Autodesk Fusion 360 part; units mm, degrees
(part 2 of 4)
sketch "Sketch1 (2)" plane through (0, -3.5, 0) normal (0, -1, 0) x (1, 0, 0) in component "Bay Cover"
  line L0 (0, -59.2) -> (2.1078, -61.3078)
  line L1 (2.1078, -61.3078) -> (5.9078, -61.3078)
  line L2 (5.9078, -61.3078) -> (9.8, -65.2)
  line L3 (9.8, -65.2) -> (18.2, -65.2)
  line L4 (18.2, -65.2) -> (23.2, -60.2)
  line L5 (23.2, -60.2) -> (87.3, -60.2)
  line L6 (87.3, -60.2) -> (92.3, -65.2)
  line L7 (92.3, -65.2) -> (100.7, -65.2)
  line L8 (100.7, -65.2) -> (108.2, -57.7)
  line L9 (108.2, -57.7) -> (108.2, 57.7)
  line L10 (108.2, 57.7) -> (100.7, 65.2)
  line L11 (100.7, 65.2) -> (92.3, 65.2)
  line L12 (92.3, 65.2) -> (87.3, 60.2)
  line L13 (87.3, 60.2) -> (23.2, 60.2)
  line L14 (23.2, 60.2) -> (18.2, 65.2)
  line L15 (18.2, 65.2) -> (9.8, 65.2)
  line L16 (9.8, 65.2) -> (5.9078, 61.3078)
  line L17 (5.9078, 61.3078) -> (2.1078, 61.3078)
  line L18 (2.1078, 61.3078) -> (0, 59.2)
  line L19 (0, 59.2) -> (0, 55.2)
  line L20 (0, 55.2) -> (4.8, 55.2)
  line L21 (4.8, 55.2) -> (4.8, 57.3078)
  line L22 (4.8, 57.3078) -> (9.5424, 55.2)
  line L23 (9.5424, 55.2) -> (100.0828, 55.2)
  line L24 (100.0828, 55.2) -> (103.2, 52.0828)
  line L25 (103.2, 52.0828) -> (103.2, -52.0828)
  line L26 (103.2, -52.0828) -> (100.0828, -55.2)
  line L27 (100.0828, -55.2) -> (9.5424, -55.2)
  line L28 (9.5424, -55.2) -> (4.8, -57.3078)
  line L29 (4.8, -57.3078) -> (4.8, -55.2)
  line L30 (4.8, -55.2) -> (0, -55.2)
  line L31 (0, -55.2) -> (0, -59.2)
  circle A0 centre (14, -60.2) radius 2.25
  circle A1 centre (96.5, -60.2) radius 2.25
  circle A2 centre (14, 60.2) radius 2.25
  circle A3 centre (96.5, 60.2) radius 2.25
  line L32 (4.8, 55.2) -> (0, 55.2)
  line L33 (0, 55.2) -> (0, 52)
  line L34 (0, 52) -> (100, 52)
  line L35 (100, 52) -> (100, -52)
  line L36 (100, -52) -> (0, -52)
  line L37 (0, -52) -> (0, -55.2)
  line L38 (0, -55.2) -> (4.8, -55.2)
  line L39 (4.8, -55.2) -> (4.8, -57.3078)
  line L40 (4.8, -57.3078) -> (9.5424, -55.2)
  line L41 (9.5424, -55.2) -> (100.0828, -55.2)
  line L42 (100.0828, -55.2) -> (103.2, -52.0828)
  line L43 (103.2, -52.0828) -> (103.2, 52.0828)
  line L44 (103.2, 52.0828) -> (100.0828, 55.2)
  line L45 (100.0828, 55.2) -> (9.5424, 55.2)
  line L46 (9.5424, 55.2) -> (4.8, 57.3078)
  line L47 (4.8, 57.3078) -> (4.8, 55.2)
extrude "Extrude1''''" add sketch "Sketch1 (2)" along normal blind 2 separate body makes body 5 in component "Bay Cover"
sketch "Sketch1 (3)" plane through (0, -5.5, 0) normal (0, -1, 0) x (1, 0, 0) in component "Spacer 40 mm"
  circle A0 centre (96.5, -60.2) radius 2.25
  circle A1 centre (14, -60.2) radius 2.25
  circle A2 centre (96.5, 60.2) radius 2.25
  circle A3 centre (14, 60.2) radius 2.25
  line L0 (0, -52) -> (0, -59.2)
  line L1 (0, -59.2) -> (2.1078, -61.3078)
  line L2 (2.1078, -61.3078) -> (5.9078, -61.3078)
  line L3 (5.9078, -61.3078) -> (9.8, -65.2)
  line L4 (9.8, -65.2) -> (18.2, -65.2)
  line L5 (18.2, -65.2) -> (23.2, -60.2)
  line L6 (23.2, -60.2) -> (87.3, -60.2)
  line L7 (87.3, -60.2) -> (92.3, -65.2)
  line L8 (92.3, -65.2) -> (100.7, -65.2)
  line L9 (100.7, -65.2) -> (108.2, -57.7)
  line L10 (108.2, -57.7) -> (108.2, 57.7)
  line L11 (108.2, 57.7) -> (100.7, 65.2)
  line L12 (100.7, 65.2) -> (92.3, 65.2)
  line L13 (92.3, 65.2) -> (87.3, 60.2)
  line L14 (87.3, 60.2) -> (23.2, 60.2)
  line L15 (23.2, 60.2) -> (18.2, 65.2)
  line L16 (18.2, 65.2) -> (9.8, 65.2)
  line L17 (9.8, 65.2) -> (5.9078, 61.3078)
  line L18 (5.9078, 61.3078) -> (2.1078, 61.3078)
  line L19 (2.1078, 61.3078) -> (0, 59.2)
  line L20 (0, 59.2) -> (0, 52)
  line L21 (0, 52) -> (100, 52)
  line L22 (100, 52) -> (100, -52)
  line L23 (100, -52) -> (0, -52)
  circle A4 centre (14, 60.2) radius 2.25
  circle A5 centre (14, 60.2) radius 4.25
  dimension "d114" = 8.5
  constraint concentric A3 A4
  constraint concentric A4 A5
  measures "d114" diameter of A5
extrude "Extrude1'''''" add sketch "Sketch1 (3)" along normal blind 40 separate body contours A5 makes body 6 in component "Spacer 40 mm"
sketch "Sketch2" plane through (0, -5.5, 0) normal (0, -1, 0) x (1, 0, 0) in component "Spacer 40 mm"
  circle A0 centre (96.5, -60.2) radius 2.25
  circle A1 centre (14, -60.2) radius 2.25
  circle A2 centre (96.5, 60.2) radius 2.25
  circle A3 centre (14, 60.2) radius 2.25
  line L0 (0, -52) -> (0, -59.2)
  line L1 (0, -59.2) -> (2.1078, -61.3078)
  line L2 (2.1078, -61.3078) -> (5.9078, -61.3078)
  line L3 (5.9078, -61.3078) -> (9.8, -65.2)
  line L4 (9.8, -65.2) -> (18.2, -65.2)
  line L5 (18.2, -65.2) -> (23.2, -60.2)
  line L6 (23.2, -60.2) -> (87.3, -60.2)
  line L7 (87.3, -60.2) -> (92.3, -65.2)
  line L8 (92.3, -65.2) -> (100.7, -65.2)
  line L9 (100.7, -65.2) -> (108.2, -57.7)
  line L10 (108.2, -57.7) -> (108.2, 57.7)
  line L11 (108.2, 57.7) -> (100.7, 65.2)
  line L12 (100.7, 65.2) -> (92.3, 65.2)
  line L13 (92.3, 65.2) -> (87.3, 60.2)
  line L14 (87.3, 60.2) -> (23.2, 60.2)
  line L15 (23.2, 60.2) -> (18.2, 65.2)
  line L16 (18.2, 65.2) -> (9.8, 65.2)
  line L17 (9.8, 65.2) -> (5.9078, 61.3078)
  line L18 (5.9078, 61.3078) -> (2.1078, 61.3078)
  line L19 (2.1078, 61.3078) -> (0, 59.2)
  line L20 (0, 59.2) -> (0, 52)
  line L21 (0, 52) -> (100, 52)
  line L22 (100, 52) -> (100, -52)
  line L23 (100, -52) -> (0, -52)
  line L24 (14, 60.2) -> (14, 65.2) construction
  circle A4 centre (14, 60.2) radius 4.25 construction
  line L25 (14, 65.2) -> (14, 64.45) construction
  dimension "d117" = 0.75
  constraint coincident A3.centre L24.start
  constraint midpoint L16 L24.end
  constraint coincident A4 L25.end
  constraint coincident L24 L25.end
  measures "d117" distance of L24.end L25.end
sketch "More Fill Ins" plane through (0, 7, 0) normal (0, 1, 0) x (-1, 0, 0) in component "End Frame A"
  line L0 (-26.9133, 50.2) -> (-55.25, 8.8457)
  line L1 (-55.25, 8.8457) -> (-83.5867, 50.2)
  line L2 (-83.5867, 50.2) -> (-26.9133, 50.2)
  line L3 (-61.3112, 0) -> (-95.709, -50.2)
  line L4 (-95.709, -50.2) -> (-98.2, -50.2)
  line L5 (-98.2, -50.2) -> (-98.2, 50.2)
  line L6 (-98.2, 50.2) -> (-95.709, 50.2)
  line L7 (-95.709, 50.2) -> (-61.3112, 0)
  line L8 (-14.791, -50.2) -> (-49.1888, 0)
  line L9 (-49.1888, 0) -> (-14.791, 50.2)
  line L10 (-14.791, 50.2) -> (-12.3, 50.2)
  line L11 (-12.3, 50.2) -> (-12.3, -50.2)
  line L12 (-12.3, -50.2) -> (-14.791, -50.2)
  line L13 (-26.9133, -50.2) -> (-83.5867, -50.2)
  line L14 (-83.5867, -50.2) -> (-55.25, -8.8457)
  line L15 (-55.25, -8.8457) -> (-26.9133, -50.2)
  circle A0 centre (-14, -60.2) radius 1.5
  circle A1 centre (-14, 60.2) radius 1.5
  circle A2 centre (-96.5, -60.2) radius 1.5
  circle A3 centre (-96.5, 60.2) radius 1.5
  line L16 (-104.0433, 68.7355) -> (-105.0433, 67.7355)
  line L17 (-105.0433, 67.7355) -> (-105.0433, 60.8567)
  line L18 (-105.0433, 60.8567) -> (-108.2, 57.7)
  line L19 (-108.2, 57.7) -> (-108.2, -57.7)
  line L20 (-108.2, -57.7) -> (-100.7, -65.2)
  line L21 (-100.7, -65.2) -> (-92.3, -65.2)
  line L22 (-92.3, -65.2) -> (-87.3, -60.2)
  line L23 (-87.3, -60.2) -> (-23.2, -60.2)
  line L24 (-23.2, -60.2) -> (-18.2, -65.2)
  line L25 (-18.2, -65.2) -> (-9.8, -65.2)
  line L26 (-9.8, -65.2) -> (-2.3, -57.7)
  line L27 (-2.3, -57.7) -> (-2.3, 57.7)
  line L28 (-2.3, 57.7) -> (-5.4567, 60.8567)
  line L29 (-5.4567, 60.8567) -> (-5.4567, 67.7355)
  line L30 (-5.4567, 67.7355) -> (-6.4567, 68.7355)
  line L31 (-6.4567, 68.7355) -> (-8.2145, 68.7355)
  line L32 (-8.2145, 68.7355) -> (-11.75, 65.2)
  line L33 (-11.75, 65.2) -> (-16.25, 65.2)
  line L34 (-16.25, 65.2) -> (-19.7855, 68.7355)
  line L35 (-19.7855, 68.7355) -> (-21.5433, 68.7355)
  line L36 (-21.5433, 68.7355) -> (-22.5433, 67.7355)
  line L37 (-22.5433, 67.7355) -> (-22.5433, 60.8567)
  line L38 (-22.5433, 60.8567) -> (-23.2, 60.2)
  line L39 (-23.2, 60.2) -> (-87.3, 60.2)
  line L40 (-87.3, 60.2) -> (-87.9567, 60.8567)
  line L41 (-87.9567, 60.8567) -> (-87.9567, 67.7355)
  line L42 (-87.9567, 67.7355) -> (-88.9567, 68.7355)
  line L43 (-88.9567, 68.7355) -> (-90.7145, 68.7355)
  line L44 (-90.7145, 68.7355) -> (-94.25, 65.2)
  line L45 (-94.25, 65.2) -> (-98.75, 65.2)
  line L46 (-98.75, 65.2) -> (-102.2855, 68.7355)
  line L47 (-102.2855, 68.7355) -> (-104.0433, 68.7355)
  line L48 (-102.2855, 68.7355) -> (-90.7145, 68.7355)
  line L49 (-19.7855, 68.7355) -> (-8.2145, 68.7355)
  line L50 (-98.2, -45.8964) -> (-92.7601, -45.8964)
  line L51 (-17.7399, -45.8964) -> (-12.3, -45.8964)
  constraint coincident L46.end L47.start
  constraint coincident L43.end L44.start
  constraint coincident L34.end L35.start
  constraint coincident L31.end L32.start
  constraint coincident L5 L50.start
  constraint coincident L3 L50.end
  constraint perpendicular L5 L50
  constraint coincident L8 L51.start
  constraint coincident L11 L51.end
  constraint perpendicular L11 L51
extrude "Extrude8" add sketch "More Fill Ins" against normal blind 3 contours L3 L4 L5 L50 | L8 L11 L12 L51 | L44 L45 L46 L48 | L32 L33 L34 L49 bodies 3 in component "End Frame A"
extrude "Extrude3''" add 1 faces at (14.3152, 9, 61.4563) along direction (0, 1, 0) blind 1 on bodies 4 bodies 4 in component "Standoff for End Frame"
extrude "Extrude9" add 4 faces at (20.0096, -1, 67.1211) (102.5096, -1, 67.1211) (19.9406, -1, -53.3479) (90.5594, -1, -53.3479) along direction (0, -1, 0) blind 9 on bodies 3 bodies 3 in component "End Frame A"
ref_plane "WorkPlane1" through (14, 4, 60.2) normal (1, 0, 0) x (0, 1, 0) in component "End Frame A"
sketch "Sketch8" plane through (14, 4, 60.2) normal (1, 0, 0) x (0, 1, 0) in component "End Frame A"
  line L0 (0, -4.2) -> (0, 0)
  line L1 (0, 0) -> (-14, 0)
  line L2 (-14, 0) -> (-14, -4.2)
  line L3 (-14, 0) -> (0, 0)
  line L4 (0, -117.9) -> (0, -2.5)
  line L5 (0, -2.5) -> (3, -2.5)
  line L6 (3, -2.5) -> (3, -117.9)
  line L7 (3, -117.9) -> (0, -117.9)
  line L8 (0, -124.6) -> (0, -120.4)
  line L9 (0, -120.4) -> (-14, -120.4)
  line L10 (-14, -120.4) -> (-14, -124.6)
  line L11 (-14, -120.4) -> (0, -120.4)
  line L12 (0, -125.4) -> (0, -117.9)
  line L13 (0, -117.9) -> (3, -117.9)
  line L14 (3, -117.9) -> (3, -125.4)
  line L15 (3, -125.4) -> (0, -125.4)
  line L16 (-14, -4.2) -> (0, -9.6008)
  line L17 (-14, -124.6) -> (-11.1871, -125.4)
  line L18 (-11.1871, -125.4) -> (0, -125.4)
  line L19 (-14, -124.6) -> (-14, -123.6)
  line L20 (-14, -123.6) -> (0, -123.6)
  line L21 (0, -125.4) -> (0, -123.6)
  line L22 (-14, -4.2) -> (-14, -3.2)
  line L23 (-14, -3.2) -> (0, -3.2)
  dimension "d124" = 1
  dimension "d125" = 90
  dimension "d126" = 180
  dimension "d127" = 1
  constraint coincident L2.end L16.start
  constraint coincident L4 L16.end
  constraint coincident L10.end L17.start
  constraint coincident L12.start L15.end
  constraint perpendicular L12 L18
  constraint parallel L10 L19
  constraint coincident L12 L20.end
  constraint horizontal L23
  constraint coincident L4 L23.end
  measures "d124" distance of L10.end L19.end
  measures "d125" angle of L19 L20
  measures "d126" angle of L21 L22
  measures "d127" distance of L2.end L22.end
extrude "Extrude10" add sketch "Sketch8" along normal mid plane 2 contours L0 L2 L4 L16 L22 L23 | L8 L10 L12 L17 L18 L19 L20 L21 bodies 3 in component "End Frame A"
ref_plane "WorkPlane2" through (96.5, -10, -60.2) normal (-1, 0, 0) x (0, -1, 0) in component "End Frame A"
sketch "Sketch9" plane through (96.5, -10, -60.2) normal (-1, 0, 0) x (0, 1, 0) in component "End Frame A"
  line L0 (14, -116.3208) -> (0, -116.3208)
  line L1 (0, -116.3208) -> (0, -116.2)
  line L2 (0, -116.2) -> (14, -110.7992)
  line L3 (14, -110.7992) -> (14, -116.3208)
  line L4 (14, 4.0792) -> (0, 4.0792)
  line L5 (0, 4.0792) -> (0, 4.2)
  line L6 (0, 4.2) -> (2.8129, 5)
  line L7 (2.8129, 5) -> (14, 5)
  line L8 (14, 5) -> (14, 4.0792)
  line L9 (14, 5) -> (2.8129, 5)
  line L10 (2.8129, 5) -> (0, 4.2)
  line L11 (0, 4.2) -> (0, 3.2)
  line L12 (0, 3.2) -> (14, 3.2)
  line L13 (14, 3.2) -> (14, 5)
  line L14 (14, -110.7992) -> (0, -116.2)
  line L15 (0, -116.2) -> (0, -117.2)
  line L16 (0, -117.2) -> (14, -117.2)
  line L17 (14, -117.2) -> (14, -110.7992)
  dimension "d130" = 1
  dimension "d131" = 1
  constraint coincident L7.end L8.start
  constraint coincident L6.end L7.start
  constraint coincident L5.end L6.start
  constraint perpendicular L4 L11
  constraint perpendicular L8 L12
  constraint perpendicular L9 L13
  constraint coincident L2.end L3.start
  constraint coincident L1.end L2.start
  constraint perpendicular L0 L15
  constraint perpendicular L3 L16
  constraint perpendicular L16 L17
  measures "d130" distance of L5.end L11.end
  measures "d131" distance of L1.end L15.end
extrude "Extrude11" add sketch "Sketch9" along normal mid plane 2 bodies 3 in component "End Frame A"
sketch "Mounts" plane through (0, -10, 0) normal (0, -1, 0) x (1, 0, 0) in component "End Frame B"
  arc A0 (97.5, 56.1208) -> (100.7, 60.2) centre (96.5, 60.2) ccw
  arc A1 (94.25, 60.2) -> (98.75, 60.2) centre (96.5, 60.2) ccw
  line L0 (88.4567, 68.2355) -> (92.3, 64.3923)
  line L1 (92.3, 64.3923) -> (92.3, 60.2)
  arc A2 (92.3, 60.2) -> (95.5, 56.1208) centre (96.5, 60.2) ccw
  line L2 (95.5, 56.1208) -> (95.5, 56)
  line L3 (95.5, 56) -> (97.5, 56)
  line L4 (97.5, 56) -> (97.5, 56.1208)
  line L5 (91.5, 57.95) -> (87.9645, 54.4145)
  line L6 (87.9645, 52.6567) -> (88.4645, 52.1567)
  line L7 (87.9645, 52.6567) -> (87.9645, 54.4145)
  line L8 (88.4645, 52.1567) -> (92.3077, 56)
  line L9 (91.5, 57.95) -> (96.5, 57.95)
  line L10 (91.5, 62.45) -> (96.5, 62.45)
  line L11 (88.4645, 68.2433) -> (87.9645, 67.7433)
  line L12 (87.9645, 67.7433) -> (87.9645, 65.9855)
  line L13 (87.9645, 65.9855) -> (91.5, 62.45)
  line L14 (92.3077, 64.4) -> (96.5, 64.4)
  line L15 (92.3077, 56) -> (96.5, 56)
  circle A3 centre (96.5, 60.2) radius 2.25
  circle A4 centre (96.5, 60.2) radius 4.2
  line L16 (92.3077, 64.4) -> (88.4567, 68.2355)
  circle A5 centre (14, 60.2) radius 1.5
  circle A6 centre (96.5, -60.2) radius 1.5
  line L17 (9.8077, 64.4) -> (5.9567, 68.2355)
  line L18 (5.9645, 68.2433) -> (5.4645, 67.7433)
  line L19 (5.4645, 67.7433) -> (5.4645, 65.9855)
  line L20 (5.4645, 65.9855) -> (9, 62.45)
  line L21 (9.8077, 64.4) -> (14, 64.4)
  circle A7 centre (14, 60.2) radius 4.2
  line L22 (9, 62.45) -> (14, 62.45)
  circle A8 centre (14, 60.2) radius 2.25
  line L23 (9, 57.95) -> (14, 57.95)
  line L24 (9.8077, 56) -> (14, 56)
  line L25 (5.9645, 52.1567) -> (9.8077, 56)
  line L26 (9, 57.95) -> (5.4645, 54.4145)
  line L27 (5.4645, 52.6567) -> (5.4645, 54.4145)
  line L28 (5.4645, 52.6567) -> (5.9645, 52.1567)
  line L29 (92.3077, -56) -> (88.4567, -52.1645)
  line L30 (88.4645, -52.1567) -> (87.9645, -52.6567)
  line L31 (87.9645, -52.6567) -> (87.9645, -54.4145)
  line L32 (87.9645, -54.4145) -> (91.5, -57.95)
  line L33 (92.3077, -56) -> (96.5, -56)
  circle A9 centre (96.5, -60.2) radius 4.2
  line L34 (91.5, -57.95) -> (96.5, -57.95)
  circle A10 centre (96.5, -60.2) radius 2.25
  line L35 (91.5, -62.45) -> (96.5, -62.45)
  line L36 (92.3077, -64.4) -> (96.5, -64.4)
  line L37 (88.4645, -68.2433) -> (92.3077, -64.4)
  line L38 (91.5, -62.45) -> (87.9645, -65.9855)
  line L39 (87.9645, -67.7433) -> (87.9645, -65.9855)
  line L40 (87.9645, -67.7433) -> (88.4645, -68.2433)
  line L41 (9.8077, -56) -> (5.9567, -52.1645)
  line L42 (5.9645, -52.1567) -> (5.4645, -52.6567)
  line L43 (5.4645, -52.6567) -> (5.4645, -54.4145)
  line L44 (5.4645, -54.4145) -> (9, -57.95)
  line L45 (9.8077, -56) -> (14, -56)
  circle A11 centre (14, -60.2) radius 4.2
  line L46 (9, -57.95) -> (14, -57.95)
  circle A12 centre (14, -60.2) radius 2.25
  line L47 (9, -62.45) -> (14, -62.45)
  line L48 (9.8077, -64.4) -> (14, -64.4)
  line L49 (5.9645, -68.2433) -> (9.8077, -64.4)
  line L50 (9, -62.45) -> (5.4645, -65.9855)
  line L51 (5.4645, -67.7433) -> (5.4645, -65.9855)
  line L52 (5.4645, -67.7433) -> (5.9645, -68.2433)
  dimension "d138" = -82.5
  dimension "d139" = -120.4
  constraint concentric A0 A3
  constraint coincident L1.end A4
  constraint coincident L0.start L16.end
extrude "Extrude1''''''" add sketch "Mounts" against normal blind 17 separate body contours A0 A1 A2 L9 L10 A3 A4 | L0 L1 L10 L14 A4 L16 | A2 L2 L5 L6 L7 L8 L9 L15 A4 | L0 L1 L10 L11 L12 L13 | L17 L18 L19 L20 L21 A7 L22 | A7 L22 A8 L23 | A7 L23 L24 L25 L26 L27 L28 | L29 L30 L31 L32 L33 A9 L34 | A9 L34 A10 L35 | A9 L35 L36 L37 L38 L39 L40 | L41 L42 L43 L44 L45 A11 L46 | A11 L46 A12 L47 | A11 L47 L48 L49 L50 L51 L52 picked at (13.7996, 63.7356) picked at (96.2996, -56.6644) picked at (13.7996, -63.7356) makes body 7 at (98.0845, -4.3333, 64.0897) makes body 8 at (97.3322, 1.3333, -64.3167) makes body 9 at (16.536, 1.3333, 56.852) makes body 10 at (16.536, 1.3333, -63.548) in component "End Frame B"
sketch "Base Shape (4)" plane through (0, 4, 0) normal (0, 1, 0) x (-1, 0, 0) in component "End Frame B"
  circle A0 centre (-14, 60.2) radius 2.25
  circle A1 centre (-14, -60.2) radius 2.25
  circle A2 centre (-96.5, 60.2) radius 2.25
  circle A3 centre (-96.5, -60.2) radius 2.25
  line L0 (-2.1078, -61.3078) -> (0, -59.2)
  line L1 (0, -59.2) -> (0, -52)
  line L2 (0, -52) -> (-100, -52)
  line L3 (-100, -52) -> (-100, 52)
  line L4 (-100, 52) -> (0, 52)
  line L5 (0, 52) -> (0, 59.2)
  line L6 (0, 59.2) -> (-2.1078, 61.3078)
  line L7 (-2.1078, 61.3078) -> (-5.9078, 61.3078)
  line L8 (-5.9078, 61.3078) -> (-9.8, 65.2)
  line L9 (-9.8, 65.2) -> (-18.2, 65.2)
  line L10 (-18.2, 65.2) -> (-23.2, 60.2)
  line L11 (-23.2, 60.2) -> (-87.3, 60.2)
  line L12 (-87.3, 60.2) -> (-92.3, 65.2)
  line L13 (-92.3, 65.2) -> (-100.7, 65.2)
  line L14 (-100.7, 65.2) -> (-108.2, 57.7)
  line L15 (-108.2, 57.7) -> (-108.2, -57.7)
  line L16 (-108.2, -57.7) -> (-100.7, -65.2)
  line L17 (-100.7, -65.2) -> (-92.3, -65.2)
  line L18 (-92.3, -65.2) -> (-87.3, -60.2)
  line L19 (-87.3, -60.2) -> (-23.2, -60.2)
  line L20 (-23.2, -60.2) -> (-18.2, -65.2)
  line L21 (-18.2, -65.2) -> (-9.8, -65.2)
  line L22 (-9.8, -65.2) -> (-5.9078, -61.3078)
  line L23 (-5.9078, -61.3078) -> (-2.1078, -61.3078)
  line L24 (-87.3, 60.2) -> (-92.3, 65.2)
  line L25 (-100.7, 65.2) -> (-92.3, 65.2)
  line L26 (-100.7, 65.2) -> (-108.2, 57.7)
  line L27 (-108.2, 57.7) -> (-108.2, -57.7)
  line L28 (-108.2, -57.7) -> (-100.7, -65.2)
  line L29 (-100.7, -65.2) -> (-92.3, -65.2)
  line L30 (-92.3, -65.2) -> (-87.3, -60.2)
  line L31 (-87.3, -60.2) -> (-23.2, -60.2)
  line L32 (-23.2, -60.2) -> (-18.2, -65.2)
  line L33 (-18.2, -65.2) -> (-9.8, -65.2)
  line L34 (-9.8, -65.2) -> (-7.8539, -63.2539)
  line L35 (-87.3, 60.2) -> (-23.2, 60.2)
  line L36 (-23.2, 60.2) -> (-18.2, 65.2)
  line L37 (-18.2, 65.2) -> (-9.8, 65.2)
  line L38 (-9.8, 65.2) -> (-7.8539, 63.2539)
  circle A4 centre (-96.5, 60.2) radius 2.25
  circle A5 centre (-14, 60.2) radius 2.25
  circle A6 centre (-14, -60.2) radius 2.25
  circle A7 centre (-96.5, -60.2) radius 2.25
  line L39 (-5.4645, 54.4145) -> (-9, 57.95)
  line L40 (-9, 57.95) -> (-14, 57.95)
  arc A8 (-14, 62.45) -> (-14, 57.95) centre (-14, 60.2) ccw
  line L41 (-14, 62.45) -> (-9, 62.45)
  line L42 (-9, 62.45) -> (-5.4645, 65.9855)
  line L43 (-5.4645, 65.9855) -> (-5.4645, 67.7433)
  line L44 (-5.4645, 67.7433) -> (-5.9567, 68.2355)
  line L45 (-5.9567, 68.2355) -> (-9.8077, 64.4)
  line L46 (-9.8077, 64.4) -> (-14, 64.4)
  arc A9 (-14, 64.4) -> (-14, 56) centre (-14, 60.2) ccw
  line L47 (-14, 56) -> (-9.8077, 56)
  line L48 (-9.8077, 56) -> (-5.9645, 52.1567)
  line L49 (-5.9645, 52.1567) -> (-5.4645, 52.6567)
  line L50 (-5.4645, 52.6567) -> (-5.4645, 54.4145)
  line L51 (-5.4645, -65.9855) -> (-9, -62.45)
  line L52 (-9, -62.45) -> (-14, -62.45)
  arc A10 (-14, -57.95) -> (-14, -62.45) centre (-14, -60.2) ccw
  line L53 (-14, -57.95) -> (-9, -57.95)
  line L54 (-9, -57.95) -> (-5.4645, -54.4145)
  line L55 (-5.4645, -54.4145) -> (-5.4645, -52.6567)
  line L56 (-5.4645, -52.6567) -> (-5.9567, -52.1645)
  line L57 (-5.9567, -52.1645) -> (-9.8077, -56)
  line L58 (-9.8077, -56) -> (-14, -56)
  arc A11 (-14, -56) -> (-14, -64.4) centre (-14, -60.2) ccw
  line L59 (-14, -64.4) -> (-9.8077, -64.4)
  line L60 (-9.8077, -64.4) -> (-5.9645, -68.2433)
  line L61 (-5.9645, -68.2433) -> (-5.4645, -67.7433)
  line L62 (-5.4645, -67.7433) -> (-5.4645, -65.9855)
  line L63 (-5.4645, 65.9855) -> (-5.4645, -67.7433)
  line L64 (-87.9645, -65.9855) -> (-91.5, -62.45)
  line L65 (-91.5, -62.45) -> (-96.5, -62.45)
  arc A12 (-96.5, -57.95) -> (-96.5, -62.45) centre (-96.5, -60.2) ccw
  line L66 (-96.5, -57.95) -> (-91.5, -57.95)
  line L67 (-91.5, -57.95) -> (-87.9645, -54.4145)
  line L68 (-87.9645, -54.4145) -> (-87.9645, -52.6567)
  line L69 (-87.9645, -52.6567) -> (-88.4567, -52.1645)
  line L70 (-88.4567, -52.1645) -> (-92.3077, -56)
  line L71 (-92.3077, -56) -> (-96.5, -56)
  arc A13 (-96.5, -56) -> (-96.5, -64.4) centre (-96.5, -60.2) ccw
  line L72 (-96.5, -64.4) -> (-92.3077, -64.4)
  line L73 (-92.3077, -64.4) -> (-88.4645, -68.2433)
  line L74 (-88.4645, -68.2433) -> (-87.9645, -67.7433)
  line L75 (-87.9645, -67.7433) -> (-87.9645, -65.9855)
  arc A14 (-96.5, 64.4) -> (-95.5, 56.1208) centre (-96.5, 60.2) ccw
  line L76 (-95.5, 56.1208) -> (-95.5, 56)
  line L77 (-95.5, 56) -> (-92.3077, 56)
  line L78 (-92.3077, 56) -> (-88.4645, 52.1567)
  line L79 (-88.4645, 52.1567) -> (-87.9645, 52.6567)
  line L80 (-87.9645, 52.6567) -> (-87.9645, 54.4145)
  line L81 (-87.9645, 54.4145) -> (-91.5, 57.95)
  line L82 (-91.5, 57.95) -> (-96.5, 57.95)
  arc A15 (-96.5, 62.45) -> (-96.5, 57.95) centre (-96.5, 60.2) ccw
  line L83 (-96.5, 62.45) -> (-91.5, 62.45)
  line L84 (-91.5, 62.45) -> (-87.9645, 65.9855)
  line L85 (-87.9645, 65.9855) -> (-87.9645, 67.7433)
  line L86 (-87.9645, 67.7433) -> (-88.4567, 68.2355)
  line L87 (-88.4567, 68.2355) -> (-92.3077, 64.4)
  line L88 (-92.3077, 64.4) -> (-96.5, 64.4)
  line L89 (-87.9645, 65.9855) -> (-87.9645, -65.9855)
  line L90 (-5.9567, 68.2355) -> (-14, 68.2355)
  line L91 (-18.2, 65.2) -> (-15.1645, 68.2355)
  line L92 (-15.1645, 68.2355) -> (-14, 68.2355)
  line L93 (-100.7, 65.2) -> (-97.6645, 68.2355)
  line L94 (-97.6645, 68.2355) -> (-88.4567, 68.2355)
  line L95 (-100.7, -65.2) -> (-97.6567, -68.2433)
  line L96 (-97.6567, -68.2433) -> (-88.4645, -68.2433)
  line L97 (-18.2, -65.2) -> (-15.1567, -68.2433)
  line L98 (-15.1567, -68.2433) -> (-5.9645, -68.2433)
  constraint coincident L11.end L12.start
  constraint coincident L12.end L13.start
  constraint coincident L13.end L14.start
  constraint coincident L14.end L15.start
  constraint coincident L15.end L16.start
  constraint coincident L16.end L17.start
  constraint coincident L17.end L18.start
  constraint coincident L18.end L19.start
  constraint coincident L19.end L20.start
  constraint coincident L20.end L21.start
  constraint coincident L21.end L22.start
  constraint midpoint L22 L34.end
  constraint coincident L10.end L11.start
  constraint coincident L9.end L10.start
  constraint coincident L8.end L9.start
  constraint midpoint L8 L38.end
  constraint concentric A2 A4
  constraint concentric A0 A5
  constraint concentric A1 A6
  constraint concentric A3 A7
  constraint coincident L42.end L43.start
  constraint coincident L61.end L62.start
  constraint coincident L84.end L85.start
  constraint coincident L64.start L75.end
  constraint coincident L44.end L45.start
  constraint perpendicular L89 L90
  constraint parallel L36 L91
  constraint parallel L90 L92
  constraint parallel L26 L93
  constraint coincident L86.end L87.start
  constraint parallel L25 L94
  constraint perpendicular L74 L95
  constraint coincident L73.end L74.start
  constraint parallel L94 L96
  constraint perpendicular L61 L97
  constraint coincident L60.end L61.start
  constraint parallel L96 L98
extrude "Extrude3'''" add sketch "Base Shape (4)" along normal blind 3 contours A0 A5 A8 | A2 A4 A15 | A1 A6 A10 | A3 A7 A12 bodies 7 8 9 10 in component "End Frame B"
extrude "Extrude2'''" add sketch "Base Shape (4)" along normal blind 3 contours A0 L7 L8 L38 A5 L39 L40 L41 L42 L63 | L7 L8 L38 L42 L63 | L4 L8 L9 L10 L11 L12 L24 L35 L36 L37 L38 L45 L46 A9 L47 L48 L49 L63 L80 L89 | L8 L9 L37 L38 L45 L90 L91 L92 | L2 L4 L63 L89 | L2 L3 L4 L89 | L2 L3 L4 L12 L13 L14 L15 L16 L17 L18 L24 L25 L26 L27 L28 L29 L30 L69 L70 L71 A13 L72 L73 A14 L76 L77 L78 L79 L87 L88 L89 | L2 L18 L19 L20 L21 L22 L30 L31 L32 L33 L34 L56 L57 L58 A11 L59 L60 L63 L68 L89 | A2 L12 L24 A4 L81 L82 L83 L84 L89 | A1 L22 L23 L34 A6 L51 L52 L53 L54 L63 | L12 L24 L84 L89 | A3 L18 L30 A7 L64 L65 L66 L67 L89 | L22 L23 L34 L51 L63 | L18 L30 L64 L89 | L12 L13 L24 L25 L87 L93 L94 | L17 L18 L29 L30 L73 L95 L96 | L21 L22 L33 L34 L60 L97 L98 bodies 7 8 9 10 in component "End Frame B"
sketch "Geometry fix" plane through (0, -10, 0) normal (0, -1, 0) x (1, 0, 0) in component "End Frame B"
  arc A0 (95.5, 56.1208) -> (96.5, 64.4) centre (96.5, 60.2) ccw
  line L0 (96.5, 64.4) -> (92.3077, 64.4)
  line L1 (92.3077, 64.4) -> (88.4567, 68.2355)
  line L2 (88.4567, 68.2355) -> (87.9645, 67.7433)
  line L3 (87.9645, 67.7433) -> (87.9645, 65.9855)
  line L4 (87.9645, 65.9855) -> (91.5, 62.45)
  line L5 (91.5, 62.45) -> (96.5, 62.45)
  arc A1 (96.5, 57.95) -> (96.5, 62.45) centre (96.5, 60.2) ccw
  line L6 (96.5, 57.95) -> (91.5, 57.95)
  line L7 (91.5, 57.95) -> (87.9645, 54.4145)
  line L8 (87.9645, 54.4145) -> (87.9645, 52.6567)
  line L9 (87.9645, 52.6567) -> (88.4645, 52.1567)
  line L10 (88.4645, 52.1567) -> (92.3077, 56)
  line L11 (92.3077, 56) -> (95.5, 56)
  line L12 (95.5, 56) -> (95.5, 56.1208)
  line L13 (95.5, 56) -> (96.5, 56)
  constraint coincident L11.end L12.start
  constraint coincident A0 L13.end
  constraint tangent A0 L13
extrude "Extrude4''" add sketch "Geometry fix" against normal blind 14 contours A0 L12 L13 bodies 7 in component "End Frame B"
sketch "Geometry fix (1)" plane through (0, 7, 0) normal (0, 1, 0) x (-1, 0, 0) in component "End Frame B"
  line L0 (-5.4645, -67.7433) -> (-5.4645, 67.7433)
  line L1 (-5.4645, 67.7433) -> (-5.9567, 68.2355)
  line L2 (-5.9567, 68.2355) -> (-15.1645, 68.2355)
  line L3 (-15.1645, 68.2355) -> (-23.2, 60.2)
  line L4 (-23.2, 60.2) -> (-87.3, 60.2)
  line L5 (-87.3, 60.2) -> (-87.9645, 60.8645)
  line L6 (-87.9645, 60.8645) -> (-87.9645, 67.7433)
  line L7 (-87.9645, 67.7433) -> (-88.4567, 68.2355)
  line L8 (-88.4567, 68.2355) -> (-97.6645, 68.2355)
  line L9 (-97.6645, 68.2355) -> (-108.2, 57.7)
  line L10 (-108.2, 57.7) -> (-108.2, -57.7)
  line L11 (-108.2, -57.7) -> (-97.6567, -68.2433)
  line L12 (-97.6567, -68.2433) -> (-88.4645, -68.2433)
  line L13 (-88.4645, -68.2433) -> (-87.9645, -67.7433)
  line L14 (-87.9645, -67.7433) -> (-87.9645, -60.8645)
  line L15 (-87.9645, -60.8645) -> (-87.3, -60.2)
  line L16 (-87.3, -60.2) -> (-23.2, -60.2)
  line L17 (-23.2, -60.2) -> (-15.1567, -68.2433)
  line L18 (-15.1567, -68.2433) -> (-5.9645, -68.2433)
  line L19 (-5.9645, -68.2433) -> (-5.4645, -67.7433)
  line L20 (-87.9645, 67.7433) -> (-80.4212, 60.2)
  line L21 (-87.9645, 67.7433) -> (-77.2967, 67.7433) construction
  line L22 (-87.9645, -67.7433) -> (-80.4212, -60.2)
  dimension "d148" = 45
  constraint horizontal L21
  constraint coincident L6.end L7.start
  constraint coincident L4 L20.end
  constraint coincident L13.end L14.start
  constraint coincident L16 L22.end
  constraint perpendicular L20 L22
  measures "d148" angle of L20 L21
extrude "Extrude5'" add sketch "Geometry fix (1)" against normal blind 3 contours L14 L15 L16 L22 | L4 L5 L6 L20 bodies 7 in component "End Frame B"
sketch "Cutouts" plane through (0, 4, 0) normal (0, -1, 0) x (1, 0, 0) in component "End Frame B"
  line L0 (96.5, 56) -> (92.3077, 56)
  line L1 (92.3077, 56) -> (88.4645, 52.1567)
  line L2 (88.4645, 52.1567) -> (87.9645, 52.6567)
  line L3 (87.9645, 52.6567) -> (87.9645, 54.4145)
  line L4 (87.9645, 54.4145) -> (91.5, 57.95)
  line L5 (91.5, 57.95) -> (96.5, 57.95)
  arc A0 (96.5, 57.95) -> (96.5, 62.45) centre (96.5, 60.2) ccw
  line L6 (96.5, 62.45) -> (91.5, 62.45)
  line L7 (91.5, 62.45) -> (87.9645, 65.9855)
  line L8 (87.9645, 65.9855) -> (87.9645, 67.7433)
  line L9 (87.9645, 67.7433) -> (80.4212, 60.2)
  line L10 (80.4212, 60.2) -> (23.2, 60.2)
  line L11 (23.2, 60.2) -> (15.1645, 68.2355)
  line L12 (15.1645, 68.2355) -> (5.9567, 68.2355)
  line L13 (5.9567, 68.2355) -> (9.8077, 64.4)
  line L14 (9.8077, 64.4) -> (14, 64.4)
  arc A1 (14, 56) -> (14, 64.4) centre (14, 60.2) ccw
  line L15 (14, 56) -> (9.8077, 56)
  line L16 (9.8077, 56) -> (5.9645, 52.1567)
  line L17 (5.9645, 52.1567) -> (5.4645, 52.6567)
  line L18 (5.4645, 52.6567) -> (5.4645, -52.6567)
  line L19 (5.4645, -52.6567) -> (5.9567, -52.1645)
  line L20 (5.9567, -52.1645) -> (9.8077, -56)
  line L21 (9.8077, -56) -> (14, -56)
  arc A2 (14, -64.4) -> (14, -56) centre (14, -60.2) ccw
  line L22 (14, -64.4) -> (9.8077, -64.4)
  line L23 (9.8077, -64.4) -> (5.9645, -68.2433)
  line L24 (5.9645, -68.2433) -> (15.1567, -68.2433)
  line L25 (15.1567, -68.2433) -> (23.2, -60.2)
  line L26 (23.2, -60.2) -> (80.4212, -60.2)
  line L27 (80.4212, -60.2) -> (87.9645, -67.7433)
  line L28 (87.9645, -67.7433) -> (87.9645, -65.9855)
  line L29 (87.9645, -65.9855) -> (91.5, -62.45)
  line L30 (91.5, -62.45) -> (96.5, -62.45)
  arc A3 (96.5, -62.45) -> (96.5, -57.95) centre (96.5, -60.2) ccw
  line L31 (96.5, -57.95) -> (91.5, -57.95)
  line L32 (91.5, -57.95) -> (87.9645, -54.4145)
  line L33 (87.9645, -54.4145) -> (87.9645, -52.6567)
  line L34 (87.9645, -52.6567) -> (88.4567, -52.1645)
  line L35 (88.4567, -52.1645) -> (92.3077, -56)
  line L36 (92.3077, -56) -> (96.5, -56)
  arc A4 (96.5, -64.4) -> (96.5, -56) centre (96.5, -60.2) ccw
  line L37 (96.5, -64.4) -> (92.3077, -64.4)
  line L38 (92.3077, -64.4) -> (88.4645, -68.2433)
  line L39 (88.4645, -68.2433) -> (97.6567, -68.2433)
  line L40 (97.6567, -68.2433) -> (108.2, -57.7)
  line L41 (108.2, -57.7) -> (108.2, 57.7)
  line L42 (108.2, 57.7) -> (97.6645, 68.2355)
  line L43 (97.6645, 68.2355) -> (88.4567, 68.2355)
  line L44 (88.4567, 68.2355) -> (92.3077, 64.4)
  line L45 (92.3077, 64.4) -> (96.5, 64.4)
  arc A5 (96.5, 56) -> (96.5, 64.4) centre (96.5, 60.2) ccw
  line L46 (15.4645, 50.2) -> (98.2, 50.2)
  line L47 (98.2, 50.2) -> (98.2, -50.2)
  line L48 (98.2, -50.2) -> (15.4645, -50.2)
  line L49 (15.4645, -50.2) -> (15.4645, 50.2)
  line L50 (44.1156, 50.2) -> (44.1156, 60.2) construction
  line L51 (98.2, 16.5867) -> (108.2, 16.5867) construction
  line L52 (68.4901, -50.2) -> (68.4901, -60.2) construction
  line L53 (15.4645, -15.1536) -> (5.4645, -15.1536) construction
  line L54 (96.5, 60.2) -> (14, -60.2) construction
  line L55 (14, 60.2) -> (96.5, -60.2) construction
  line L56 (9.8754, 57.3738) -> (92.3754, -63.0262)
  line L57 (18.1246, 63.0262) -> (100.6246, -57.3738)
  line L58 (92.3754, 63.0262) -> (9.8754, -57.3738)
  line L59 (100.6246, 57.3738) -> (18.1246, -63.0262)
  dimension "d151" = 10
  dimension "d152" = 5
  dimension "d153" = -5
  dimension "d154" = 5
  dimension "d155" = -5
  constraint horizontal L46
  constraint vertical L47
  constraint horizontal L48
  constraint vertical L49
  constraint coincident L46 L50.start
  constraint coincident L10 L50.end
  constraint perpendicular L10 L50
  constraint coincident L47 L51.start
  constraint coincident L41 L51.end
  constraint perpendicular L41 L51
  constraint coincident L48 L52.start
  constraint coincident L26 L52.end
  constraint perpendicular L26 L52
  constraint coincident L49 L53.start
  constraint coincident L18 L53.end
  constraint perpendicular L18 L53
  constraint equal L50 L51
  constraint equal L51 L52
  constraint equal L52 L53
  constraint coincident A0.centre A5.centre
  constraint coincident A2.centre L54.end
  constraint coincident A1.centre L55.start
  constraint coincident A3.centre A4.centre
  measures "d151" distance of L53.start L53.end
extrude "Extrude6''" cut sketch "Cutouts" against normal blind 15 contours L46 L57 L58 | L46 L47 L48 L57 L59 | L49 L56 L58 | L48 L56 L59 bodies 7 in component "End Frame B"
sketch "Stand-off sockets" plane through (0, 7, 0) normal (0, 1, 0) x (-1, 0, 0) in component "End Frame B"
  line L0 (-26.9133, 50.2) -> (-55.25, 8.8457)
  line L1 (-55.25, 8.8457) -> (-83.5867, 50.2)
  line L2 (-83.5867, 50.2) -> (-26.9133, 50.2)
  line L3 (-61.3112, 0) -> (-92.7601, -45.8964)
  line L4 (-92.7601, -45.8964) -> (-98.2, -45.8964)
  line L5 (-98.2, -45.8964) -> (-98.2, 50.2)
  line L6 (-98.2, 50.2) -> (-95.709, 50.2)
  line L7 (-95.709, 50.2) -> (-61.3112, 0)
  line L8 (-17.7399, -45.8964) -> (-49.1888, 0)
  line L9 (-49.1888, 0) -> (-14.791, 50.2)
  line L10 (-14.791, 50.2) -> (-12.3, 50.2)
  line L11 (-12.3, 50.2) -> (-12.3, -45.8964)
  line L12 (-12.3, -45.8964) -> (-17.7399, -45.8964)
  line L13 (-26.9133, -50.2) -> (-83.5867, -50.2)
  line L14 (-83.5867, -50.2) -> (-55.25, -8.8457)
  line L15 (-55.25, -8.8457) -> (-26.9133, -50.2)
  circle A0 centre (-14, -60.2) radius 1.5
  circle A1 centre (-14, 60.2) radius 1.5
  circle A2 centre (-96.5, -60.2) radius 1.5
  circle A3 centre (-96.5, 60.2) radius 1.5
  line L16 (-104.0433, 68.7355) -> (-105.0433, 67.7355)
  line L17 (-105.0433, 67.7355) -> (-105.0433, 60.8567)
  line L18 (-105.0433, 60.8567) -> (-108.2, 57.7)
  line L19 (-108.2, 57.7) -> (-108.2, -57.7)
  line L20 (-108.2, -57.7) -> (-100.7, -65.2)
  line L21 (-100.7, -65.2) -> (-92.3, -65.2)
  line L22 (-92.3, -65.2) -> (-87.3, -60.2)
  line L23 (-87.3, -60.2) -> (-23.2, -60.2)
  line L24 (-23.2, -60.2) -> (-18.2, -65.2)
  line L25 (-18.2, -65.2) -> (-9.8, -65.2)
  line L26 (-9.8, -65.2) -> (-2.3, -57.7)
  line L27 (-2.3, -57.7) -> (-2.3, 57.7)
  line L28 (-2.3, 57.7) -> (-5.4567, 60.8567)
  line L29 (-5.4567, 60.8567) -> (-5.4567, 67.7355)
  line L30 (-5.4567, 67.7355) -> (-6.4567, 68.7355)
  line L31 (-6.4567, 68.7355) -> (-21.5433, 68.7355)
  line L32 (-21.5433, 68.7355) -> (-22.5433, 67.7355)
  line L33 (-22.5433, 67.7355) -> (-22.5433, 60.8567)
  line L34 (-22.5433, 60.8567) -> (-23.2, 60.2)
  line L35 (-23.2, 60.2) -> (-87.3, 60.2)
  line L36 (-87.3, 60.2) -> (-87.9567, 60.8567)
  line L37 (-87.9567, 60.8567) -> (-87.9567, 67.7355)
  line L38 (-87.9567, 67.7355) -> (-88.9567, 68.7355)
  line L39 (-88.9567, 68.7355) -> (-104.0433, 68.7355)
  circle A4 centre (-96.5, 60.2) radius 1.5
  circle A5 centre (-14, 60.2) radius 1.5
  circle A6 centre (-96.5, -60.2) radius 1.5
  circle A7 centre (-14, -60.2) radius 1.5
extrude "Extrude7'" cut sketch "Stand-off sockets" against normal blind 1.5 contours A0 A7 | A1 A5 | A2 A6 | A3 A4 bodies 7 in component "End Frame B"
ref_plane "WorkPlane1" through (96.5, -10, 60.2) normal (0, 0, -1) x (-1, 0, 0) in component "End Frame B"
sketch "Sketch9 (2)" plane through (96.5, -10, 60.2) normal (0, 0, -1) x (1, 0, 0) in component "End Frame B"
  line L0 (0, 0) -> (0, -14)
  line L1 (4.2, -14) -> (0, -14)
  line L2 (0, -14) -> (0, 0)
  line L3 (4.2, 0) -> (0, 0)
  line L4 (-78.3, -14) -> (-82.5, -14)
  line L5 (-82.5, -14) -> (-82.5, 0)
  line L6 (-78.3, 0) -> (-82.5, 0)
  line L7 (-82.5, 0) -> (-82.5, -14)
  line L8 (11.7, -14) -> (1.1645, -14)
  line L9 (-73.3, -14) -> (-81.3355, -14)
  line L10 (-16.0788, -14) -> (-73.3, -14)
  line L11 (-78.3, 0) -> (-79.3, 0)
  line L12 (-79.3, 0) -> (-79.3, -14)
  line L13 (-78.3, 0) -> (-68.4971, -14)
  line L14 (-79.3, -14) -> (-68.4971, -14)
  line L15 (4.2, 0) -> (3.2, 0)
  line L16 (3.2, 0) -> (3.2, -14)
  line L17 (3.2, -14) -> (11.7, -14)
  line L18 (11.7, -14) -> (4.2, 0)
  dimension "d160" = 1
  dimension "d161" = 145
  dimension "d162" = 1
  constraint coincident L6.start L11.start
  constraint parallel L6 L11
  constraint vertical L12
  constraint coincident L4 L12.end
  constraint coincident L10 L13.end
  constraint coincident L3.start L15.start
  constraint perpendicular L0 L15
  constraint vertical L16
  constraint coincident L1 L16.end
  constraint coincident L8.start L17.end
  measures "d160" distance of L6.start L11.end
  measures "d161" angle of L12 L13
  measures "d162" distance of L3.start L15.end
extrude "Extrude8'" add sketch "Sketch9 (2)" along normal mid plane 2 contours L1 L3 L8 L15 L16 L17 L18 | L4 L6 L9 L10 L11 L12 L13 L14 bodies 7 in component "End Frame B"
sketch "Sketch11" plane through (0, 4, 0) normal (0, 1, 0) x (-1, 0, 0) in component "End Frame B"
  line L0 (-28.0029, 60.2) -> (-23.2, 60.2)
  line L1 (-23.2, 60.2) -> (-22.2, 61.2)
  line L2 (-22.2, 61.2) -> (-28.0029, 61.2)
  line L3 (-28.0029, 61.2) -> (-28.0029, 60.2)
  line L4 (-28.0029, 61.2) -> (-29.0029, 60.2)
  line L5 (-28.0029, 61.2) -> (-26.5887, 61.2) construction
  line L6 (-29.0029, 60.2) -> (-36.3615, 60.2)
  line L7 (-106.7, 59.2) -> (-104.7, 61.2)
  line L8 (-104.7, 61.2) -> (-108.2, 61.2)
  line L9 (-108.2, 61.2) -> (-108.2, 59.2)
  line L10 (-108.2, 59.2) -> (-106.7, 59.2)
  line L11 (-97.6645, 68.2355) -> (-108.2, 57.7)
  line L12 (-108.2, 59.2) -> (-108.2, 57.7)
  line L13 (-29.0029, 60.2) -> (-28.0029, 60.2)
  line L14 (0, 0) -> (-84.064, 0) construction
  line L15 (-29.0029, -60.2) -> (-28.0029, -60.2)
  line L16 (-28.0029, -61.2) -> (-29.0029, -60.2)
  line L17 (-28.0029, -61.2) -> (-28.0029, -60.2)
  line L18 (-104.7, -61.2) -> (-108.2, -61.2)
  line L19 (-97.6645, -68.2355) -> (-108.2, -57.7)
  line L20 (-108.2, -61.2) -> (-108.2, -59.2)
  line L21 (-108.2, -59.2) -> (-106.7, -59.2)
  line L22 (-108.2, -59.2) -> (-108.2, -57.7)
  line L23 (-22.2, -61.2) -> (-28.0029, -61.2)
  line L24 (-28.0029, -60.2) -> (-23.2, -60.2)
  line L25 (-23.2, -60.2) -> (-22.2, -61.2)
  dimension "d165" = 135
  dimension "d166" = 7.3586
  constraint horizontal L5
  constraint coincident L2.end L3.start
  constraint perpendicular L3 L6
  constraint coincident L9.end L10.start
  constraint coincident L11.end L12.end
  constraint coincident L0.start L3.end
  constraint perpendicular L3 L13
  constraint coincident L14.start origin
  constraint horizontal L14
  constraint symmetric L0.start L14 L15.end
  constraint symmetric L0.end L14 L24.end
  constraint symmetric L1.end L14 L23.start
  constraint symmetric L2.end L14 L16.start
  constraint symmetric L4.end L14 L15.start
  constraint symmetric L7.start L14 L21.end
  constraint symmetric L7.end L14 L18.start
  constraint symmetric L8.end L14 L18.end
  constraint symmetric L9.end L14 L20.end
  constraint symmetric L11.start L14 L19.start
  constraint symmetric L11.end L14 L19.end
  measures "d165" angle of L4 L5
  measures "d166" distance of L4.end L6.end
extrude "Extrude10'" add sketch "Sketch11" along normal blind 3 bodies 7 in component "End Frame B"
mirror "Mirror1" about plane through (0, 0, 0) normal (0, 0, 1) of "Extrude8'" in component "End Frame B"
sketch "Sketch1 (4)" plane through (0, -45.5, 0) normal (0, -1, 0) x (1, 0, 0) in component "Spacer 35 mm"
  circle A0 centre (14, 60.2) radius 2.25
  circle A1 centre (14, 60.2) radius 4.25
extrude "Extrude1'''''''" add sketch "Sketch1 (4)" against normal blind 35 separate body makes body 11 in component "Spacer 35 mm"
extrude "Extrude7''" add 1 faces at (71.6667, 0, 16.6667) along direction (0, -1, 0) blind 0.5 on bodies 1 bodies 1 in component "Card Plate"
sketch "Raspberry Pi 4" plane through (0, -0.5, 0) normal (0, -1, 0) x (1, 0, 0) in component "Card Plate"
  line L0 (100, 52) -> (15, 52)
  line L1 (15, 52) -> (15, 50)
  line L2 (15, 50) -> (0, 50)
  line L3 (0, 50) -> (0, -50)
  line L4 (0, -50) -> (15, -50)
  line L5 (15, -50) -> (15, -52)
  line L6 (15, -52) -> (100, -52)
  line L7 (100, -52) -> (100, 52)
  line L8 (0, 28) -> (85, 28) construction
  line L9 (85, 28) -> (85, -28) construction
  line L10 (85, -28) -> (0, -28) construction
  line L11 (0, -28) -> (0, 28) construction
  line L12 (22.6166, 28) -> (22.6166, 52) construction
  line L13 (22.6166, -28) -> (22.6166, -52) construction
  circle A0 centre (23.5, 24.5) radius 1.35
  circle A1 centre (81.5, 24.5) radius 1.35
  circle A2 centre (23.5, -24.5) radius 1.35
  circle A3 centre (81.5, -24.5) radius 1.35
  line L14 (23.5, 24.5) -> (81.5, 24.5) construction
  line L15 (81.5, 24.5) -> (81.5, -24.5) construction
  line L16 (81.5, -24.5) -> (23.5, -24.5) construction
  line L17 (23.5, -24.5) -> (23.5, 24.5) construction
  line L18 (35.5285, 24.5) -> (35.5285, 28) construction
  line L19 (37.1428, -24.5) -> (37.1428, -28) construction
  dimension "d177" = 85
  dimension "d178" = 56
  dimension "d179" = 2.7
  dimension "d180" = 2.7
  dimension "d181" = 2.7
  dimension "d182" = 2.7
  dimension "d183" = 58
  dimension "d184" = 49
  dimension "d185" = 3.5
  dimension "d186" = 3.5
  constraint horizontal L8
  constraint vertical L9
  constraint horizontal L10
  constraint vertical L11
  constraint coincident L8 L12.start
  constraint coincident L0 L12.end
  constraint perpendicular L0 L12
  constraint coincident L10 L13.start
  constraint coincident L6 L13.end
  constraint perpendicular L6 L13
  constraint equal L12 L13
  constraint collinear L3 L11
  constraint coincident A0.centre L14.start
  constraint coincident A1.centre L14.end
  constraint coincident A3.centre L15.end
  constraint vertical L15
  constraint coincident A2.centre L16.end
  constraint vertical L17
  constraint horizontal L14
  constraint horizontal L16
  constraint coincident L14 L18.start
  constraint coincident L8 L18.end
  constraint perpendicular L8 L18
  constraint coincident L16 L19.start
  constraint coincident L10 L19.end
  constraint perpendicular L10 L19
  measures "d177" distance of L8.start L8.end
  measures "d178" distance of L8.start L10.end
  measures "d179" diameter of A0
  measures "d180" diameter of A1
  measures "d181" diameter of A2
  measures "d182" diameter of A3
  measures "d183" distance of A0.centre A1.centre
  measures "d184" distance of A0.centre A2.centre
  measures "d185" distance of L19.start L19.end
  measures "d186" distance of L9 A3.centre
extrude "Extrude8''" cut sketch "Raspberry Pi 4" against normal blind 7 contours A0 | A1 | A2 | A3 bodies 1 in component "Card Plate"
sketch "Jetson Xavier NX" plane through (0, -0.5, 0) normal (0, -1, 0) x (1, 0, 0) in component "Card Plate"
  circle A0 centre (81.5, 24.5) radius 1.35
  circle A1 centre (81.5, -24.5) radius 1.35
  circle A2 centre (23.5, 24.5) radius 1.35
  circle A3 centre (23.5, -24.5) radius 1.35
  line L0 (100, 52) -> (15, 52)
  line L1 (15, 52) -> (15, 50)
  line L2 (15, 50) -> (0, 50)
  line L3 (0, 50) -> (0, -50)
  line L4 (0, -50) -> (15, -50)
  line L5 (15, -50) -> (15, -52)
  line L6 (15, -52) -> (100, -52)
  line L7 (100, -52) -> (100, 52)
  line L8 (0, 50) -> (79, 50) construction
  line L9 (79, 50) -> (79, -50) construction
  line L10 (79, -50) -> (0, -50) construction
  line L11 (0, -50) -> (0, 50) construction
  line L12 (29.1739, 50) -> (29.1739, 52) construction
  line L13 (30.7023, -50) -> (30.7023, -52) construction
  circle A4 centre (17, 46) radius 1.35
  circle A5 centre (75, 46) radius 1.35
  circle A6 centre (75, -46) radius 1.35
  circle A7 centre (17, -46) radius 1.35
  line L14 (75, 46) -> (17, 46) construction
  line L15 (17, 46) -> (17, -46) construction
  line L16 (17, -46) -> (75, -46) construction
  line L17 (75, -46) -> (75, 46) construction
  dimension "d189" = 79
  dimension "d190" = 100
  dimension "d191" = 2.7
  dimension "d192" = 2.7
  dimension "d193" = 2.7
  dimension "d194" = 2.7
  dimension "d195" = 58
  dimension "d196" = 92
  dimension "d197" = 4
  dimension "d198" = 4
  constraint horizontal L8
  constraint vertical L9
  constraint horizontal L10
  constraint vertical L11
  constraint coincident L8 L12.start
  constraint coincident L0 L12.end
  constraint perpendicular L0 L12
  constraint coincident L10 L13.start
  constraint coincident L6 L13.end
  constraint perpendicular L6 L13
  constraint equal L12 L13
  constraint collinear L3 L11
  constraint coincident A5.centre L14.start
  constraint coincident A4.centre L14.end
  constraint coincident A7.centre L15.end
  constraint vertical L15
  constraint coincident A6.centre L16.end
  constraint perpendicular L15 L16
  constraint perpendicular L16 L17
  constraint horizontal L14
  measures "d189" distance of L2.end L8.end
  measures "d190" distance of L2.end L3.end
  measures "d191" diameter of A4
  measures "d192" diameter of A7
  measures "d193" diameter of A6
  measures "d194" diameter of A5
  measures "d195" distance of A5.centre A4.centre
  measures "d196" distance of A5.centre A6.centre
  measures "d197" distance of L9 A5.centre
  measures "d198" distance of L10 A6.centre
extrude "Extrude9'" cut sketch "Jetson Xavier NX" against normal blind 6 contours A4 | A5 | A6 | A7 bodies 1 in component "Card Plate"
sketch "Avenger96 Extended" plane through (0, -0.5, 0) normal (0, -1, 0) x (1, 0, 0) in component "Card Plate"
  circle A0 centre (75, 46) radius 1.35
  circle A1 centre (17, -46) radius 1.35
  circle A2 centre (17, 46) radius 1.35
  circle A3 centre (75, -46) radius 1.35
  circle A4 centre (81.5, 24.5) radius 1.35
  circle A5 centre (81.5, -24.5) radius 1.35
  circle A6 centre (23.5, 24.5) radius 1.35
  circle A7 centre (23.5, -24.5) radius 1.35
  line L0 (100, 52) -> (15, 52)
  line L1 (15, 52) -> (15, 50)
  line L2 (15, 50) -> (0, 50)
  line L3 (0, 50) -> (0, -50)
  line L4 (0, -50) -> (15, -50)
  line L5 (15, -50) -> (15, -52)
  line L6 (15, -52) -> (100, -52)
  line L7 (100, -52) -> (100, 52)
  line L8 (0, 42.5) -> (100, 42.5) construction
  line L9 (100, 42.5) -> (100, -42.5) construction
  line L10 (100, -42.5) -> (0, -42.5) construction
  line L11 (0, -42.5) -> (0, 42.5) construction
  line L12 (41.855, 42.5) -> (41.855, 52) construction
  line L13 (38.6195, -42.5) -> (38.6195, -52) construction
  circle A8 centre (4, 38.5) radius 1.35
  circle A9 centre (50, 38.5) radius 1.35
  circle A10 centre (50, -38.5) radius 1.35
  circle A11 centre (4, -38.5) radius 1.35
  circle A12 centre (81.5, -38.5) radius 1.35
  circle A13 centre (81.5, 38.5) radius 1.35
  line L14 (4, 38.5) -> (50, 38.5) construction
  line L15 (50, 38.5) -> (81.5, 38.5) construction
  line L16 (81.5, 38.5) -> (81.5, -38.5) construction
  line L17 (81.5, -38.5) -> (50, -38.5) construction
  line L18 (50, -38.5) -> (4, -38.5) construction
  line L19 (4, -38.5) -> (4, 38.5) construction
  line L20 (50, 38.5) -> (50, -38.5) construction
  dimension "d201" = 100
  dimension "d202" = 85
  dimension "d203" = 2.7
  dimension "d204" = 2.7
  dimension "d205" = 2.7
  dimension "d206" = 2.7
  dimension "d207" = 2.7
  dimension "d208" = 2.7
  dimension "d209" = 4
  dimension "d210" = 4
  dimension "d211" = 46
  dimension "d212" = 31.5
  dimension "d213" = 4
  constraint horizontal L8
  constraint vertical L9
  constraint horizontal L10
  constraint vertical L11
  constraint collinear L3 L11
  constraint coincident L8 L12.start
  constraint coincident L0 L12.end
  constraint perpendicular L0 L12
  constraint coincident L10 L13.start
  constraint coincident L6 L13.end
  constraint perpendicular L6 L13
  constraint equal L12 L13
  constraint coincident A8.centre L14.start
  constraint coincident A9.centre L14.end
  constraint coincident A13.centre L15.end
  constraint horizontal L15
  constraint coincident A12.centre L16.end
  constraint coincident A10.centre L17.end
  constraint coincident A11.centre L18.end
  constraint vertical L19
  constraint vertical L20
  constraint vertical L16
  constraint horizontal L17
  constraint horizontal L14
  constraint horizontal L18
  measures "d201" distance of L8.start L8.end
  measures "d202" distance of L8.start L10.end
  measures "d203" diameter of A8
  measures "d204" diameter of A9
  measures "d205" diameter of A13
  measures "d206" diameter of A11
  measures "d207" diameter of A10
  measures "d208" diameter of A12
  measures "d209" distance of L8 A8.centre
  measures "d210" distance of L11 A11.centre
  measures "d211" distance of A10.centre A11.centre
  measures "d212" distance of A12.centre A10.centre
  measures "d213" distance of L10 A11.centre
extrude "Extrude10''" cut sketch "Avenger96 Extended" against normal blind 17 contours A8 | A9 | A10 | A11 | A12 | A13 bodies 1 in component "Card Plate"
sketch "Avenger96 Consumer" plane through (0, -0.5, 0) normal (0, -1, 0) x (1, 0, 0) in component "Card Plate"
  circle A0 centre (4, -38.5) radius 1.35
  circle A1 centre (4, 38.5) radius 1.35
  circle A2 centre (50, -38.5) radius 1.35
  circle A3 centre (81.5, 38.5) radius 1.35
  circle A4 centre (50, 38.5) radius 1.35
  circle A5 centre (81.5, -38.5) radius 1.35
  circle A6 centre (75, 46) radius 1.35
  circle A7 centre (17, -46) radius 1.35
  circle A8 centre (17, 46) radius 1.35
  circle A9 centre (75, -46) radius 1.35
  circle A10 centre (81.5, 24.5) radius 1.35
  circle A11 centre (81.5, -24.5) radius 1.35
  circle A12 centre (23.5, 24.5) radius 1.35
  circle A13 centre (23.5, -24.5) radius 1.35
  line L0 (100, 52) -> (15, 52)
  line L1 (15, 52) -> (15, 50)
  line L2 (15, 50) -> (0, 50)
  line L3 (0, 50) -> (0, -50)
  line L4 (0, -50) -> (15, -50)
  line L5 (15, -50) -> (15, -52)
  line L6 (15, -52) -> (100, -52)
  line L7 (100, -52) -> (100, 52)
  circle A14 centre (18.5, 38.5) radius 1.35
  circle A15 centre (18.5, -38.5) radius 1.35
  line L8 (4, 38.5) -> (18.5, 38.5) construction
  line L9 (18.5, -38.5) -> (18.5, 38.5) construction
  line L10 (18.5, -38.5) -> (4, -38.5) construction
  dimension "d216" = 2.7
  dimension "d217" = 2.7
  dimension "d219" = 18.5
  constraint coincident A1.centre L8.start
  constraint coincident A14.centre L8.end
  constraint coincident A15.centre L9.start
  constraint horizontal L8
  constraint vertical L9
  constraint coincident A0.centre L10.end
  constraint horizontal L10
  measures "d216" diameter of A14
  measures "d217" diameter of A15
  measures "d219" distance of L3 L9
extrude "Extrude11'" cut sketch "Avenger96 Consumer" against normal blind 24 contours A14 | A15 bodies 1 in component "Card Plate"